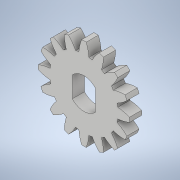
# Autodesk Inventor part: Pinion
Saved by Autodesk Inventor 2020.1 (Build 241239000, 239)
## iProperties
Created: 2019-10-24
Part Number: Pinion
Material: Generic
Document SubType Name: Modeling
Designer: ajtan
Density: 1 g/cm^3
Appearance: Default
Author: ajtan
Autodesk Inventor part; units mm, degrees
ref_plane "YZ Plane" through (0, 0, 0) normal (1, 0, 0) x (0, 1, 0)
ref_plane "XZ Plane" through (0, 0, 0) normal (0, 1, 0) x (-1, 0, 0)
ref_plane "XY Plane" through (0, 0, 0) normal (0, 0, 1) x (1, 0, 0)
sketch "Sketch3" plane through (0, 0, 0) normal (0, 0, 1) x (1, 0, 0)
  arc A0 (12.7932, -14.1151) -> (14.1151, -12.7932) centre (0, 0) ccw
  arc A1 (14.1151, -12.7932) -> (11.4758, -8.5111) centre (-0.2655, -18.7022) ccw
  arc A2 (11.4758, -8.5111) -> (12.2548, -7.3452) centre (0, 0) ccw
  arc A3 (12.2548, -7.3452) -> (17.221, -8.1449) centre (17.177, 7.4023) ccw
  arc A4 (17.221, -8.1449) -> (17.9364, -6.4178) centre (0, 0) ccw
  arc A5 (17.9364, -6.4178) -> (13.8593, -3.4716) centre (6.9118, -17.3802) ccw
  arc A6 (13.8593, -3.4716) -> (14.1329, -2.0964) centre (0, 0) ccw
  arc A7 (14.1329, -2.0964) -> (19.0271, -0.9347) centre (13.0367, 13.4122) ccw
  arc A8 (19.0271, -0.9347) -> (19.0271, 0.9347) centre (0, 0) ccw
  arc A9 (19.0271, 0.9347) -> (14.1329, 2.0964) centre (13.0367, -13.4122) ccw
  arc A10 (14.1329, 2.0964) -> (13.8593, 3.4716) centre (0, 0) ccw
  arc A11 (13.8593, 3.4716) -> (17.9364, 6.4178) centre (6.9118, 17.3802) ccw
  arc A12 (17.9364, 6.4178) -> (17.221, 8.1449) centre (0, 0) ccw
  arc A13 (17.221, 8.1449) -> (12.2548, 7.3452) centre (17.177, -7.4023) ccw
  arc A14 (12.2548, 7.3452) -> (11.4758, 8.5111) centre (0, 0) ccw
  arc A15 (11.4758, 8.5111) -> (14.1151, 12.7932) centre (-0.2655, 18.7022) ccw
  arc A16 (14.1151, 12.7932) -> (12.7932, 14.1151) centre (0, 0) ccw
  arc A17 (12.7932, 14.1151) -> (8.5111, 11.4758) centre (18.7022, -0.2655) ccw
  arc A18 (8.5111, 11.4758) -> (7.3452, 12.2548) centre (0, 0) ccw
  arc A19 (7.3452, 12.2548) -> (8.1449, 17.221) centre (-7.4023, 17.177) ccw
  arc A20 (8.1449, 17.221) -> (6.4178, 17.9364) centre (0, 0) ccw
  arc A21 (6.4178, 17.9364) -> (3.4716, 13.8593) centre (17.3802, 6.9118) ccw
  arc A22 (3.4716, 13.8593) -> (2.0964, 14.1329) centre (0, 0) ccw
  arc A23 (2.0964, 14.1329) -> (0.9347, 19.0271) centre (-13.4122, 13.0367) ccw
  arc A24 (0.9347, 19.0271) -> (-0.9347, 19.0271) centre (0, 0) ccw
  arc A25 (-0.9347, 19.0271) -> (-2.0964, 14.1329) centre (13.4122, 13.0367) ccw
  arc A26 (-2.0964, 14.1329) -> (-3.4716, 13.8593) centre (0, 0) ccw
  arc A27 (-3.4716, 13.8593) -> (-6.4178, 17.9364) centre (-17.3802, 6.9118) ccw
  arc A28 (-6.4178, 17.9364) -> (-8.1449, 17.221) centre (0, 0) ccw
  arc A29 (-8.1449, 17.221) -> (-7.3452, 12.2548) centre (7.4023, 17.177) ccw
  arc A30 (-7.3452, 12.2548) -> (-8.5111, 11.4758) centre (0, 0) ccw
  arc A31 (-8.5111, 11.4758) -> (-12.7932, 14.1151) centre (-18.7022, -0.2655) ccw
  arc A32 (-12.7932, 14.1151) -> (-14.1151, 12.7932) centre (0, 0) ccw
  arc A33 (-14.1151, 12.7932) -> (-11.4758, 8.5111) centre (0.2655, 18.7022) ccw
  arc A34 (-11.4758, 8.5111) -> (-12.2548, 7.3452) centre (0, 0) ccw
  arc A35 (-12.2548, 7.3452) -> (-17.221, 8.1449) centre (-17.177, -7.4023) ccw
  arc A36 (-17.221, 8.1449) -> (-17.9364, 6.4178) centre (0, 0) ccw
  arc A37 (-17.9364, 6.4178) -> (-13.8593, 3.4716) centre (-6.9118, 17.3802) ccw
  arc A38 (-13.8593, 3.4716) -> (-14.1329, 2.0964) centre (0, 0) ccw
  arc A39 (-14.1329, 2.0964) -> (-19.0271, 0.9347) centre (-13.0367, -13.4122) ccw
  arc A40 (-19.0271, 0.9347) -> (-19.0271, -0.9347) centre (0, 0) ccw
  arc A41 (-19.0271, -0.9347) -> (-14.1329, -2.0964) centre (-13.0367, 13.4122) ccw
  arc A42 (-14.1329, -2.0964) -> (-13.8593, -3.4716) centre (0, 0) ccw
  arc A43 (-13.8593, -3.4716) -> (-17.9364, -6.4178) centre (-6.9118, -17.3802) ccw
  arc A44 (-17.9364, -6.4178) -> (-17.221, -8.1449) centre (0, 0) ccw
  arc A45 (-17.221, -8.1449) -> (-12.2548, -7.3452) centre (-17.177, 7.4023) ccw
  arc A46 (-12.2548, -7.3452) -> (-11.4758, -8.5111) centre (0, 0) ccw
  arc A47 (-11.4758, -8.5111) -> (-14.1151, -12.7932) centre (0.2655, -18.7022) ccw
  arc A48 (-14.1151, -12.7932) -> (-12.7932, -14.1151) centre (0, 0) ccw
  arc A49 (-12.7932, -14.1151) -> (-8.5111, -11.4758) centre (-18.7022, 0.2655) ccw
  arc A50 (-8.5111, -11.4758) -> (-7.3452, -12.2548) centre (0, 0) ccw
  arc A51 (-7.3452, -12.2548) -> (-8.1449, -17.221) centre (7.4023, -17.177) ccw
  arc A52 (-8.1449, -17.221) -> (-6.4178, -17.9364) centre (0, 0) ccw
  arc A53 (-6.4178, -17.9364) -> (-3.4716, -13.8593) centre (-17.3802, -6.9118) ccw
  arc A54 (-3.4716, -13.8593) -> (-2.0964, -14.1329) centre (0, 0) ccw
  arc A55 (-2.0964, -14.1329) -> (-0.9347, -19.0271) centre (13.4122, -13.0367) ccw
  arc A56 (-0.9347, -19.0271) -> (0.9347, -19.0271) centre (0, 0) ccw
  arc A57 (0.9347, -19.0271) -> (2.0964, -14.1329) centre (-13.4122, -13.0367) ccw
  arc A58 (2.0964, -14.1329) -> (3.4716, -13.8593) centre (0, 0) ccw
  arc A59 (3.4716, -13.8593) -> (6.4178, -17.9364) centre (17.3802, -6.9118) ccw
  arc A60 (6.4178, -17.9364) -> (8.1449, -17.221) centre (0, 0) ccw
  arc A61 (8.1449, -17.221) -> (7.3452, -12.2548) centre (-7.4023, -17.177) ccw
  arc A62 (7.3452, -12.2548) -> (8.5111, -11.4758) centre (0, 0) ccw
  arc A63 (8.5111, -11.4758) -> (12.7932, -14.1151) centre (18.7022, 0.2655) ccw
  circle A64 centre (0, 0) radius 16.9291 construction
  line L0 (-4.826, 4.3199) -> (-4.826, -4.3199)
  line L1 (4.826, 4.3199) -> (4.826, -4.3199)
  arc A65 (-4.826, -4.3199) -> (4.826, -4.3199) centre (0, 0) ccw
  arc A66 (4.826, 4.3199) -> (-4.826, 4.3199) centre (0, 0) ccw
  dimension "d14" = 19.05
  dimension "d15" = 33.8582
  dimension "d8" = 4.826
  dimension "d9" = 9.652
  dimension "d10" = 6.477
  dimension "d11" = 6.477
  constraints: 68 point on circle, 34 centre point, 4 end point, 2 horizontal alignment, 2 vertical, 2 vertical alignment, 93 other
  measures "d8" distance of the line from the sketch origin of L1
  measures "d9" distance between parallel lines of L0 L1
  measures "d10" radius of A66
  measures "d11" radius of A65
extrude "Extrusion2" add sketch "Sketch3" along normal blind 5.08
body "Solid2"
